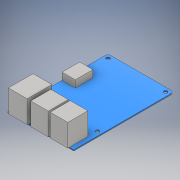
# Autodesk Inventor part: learnbotOdroid
Saved by Autodesk Inventor 2017 (Build 210142000, 142)
## iProperties
Part Number: learnbotOdroid
Material: Genérico
Document SubType Name: Modeling
Designer: rober
Density: 1 g/cm^3
Appearance: Valor por defecto
Author: rober
Autodesk Inventor part; units mm, degrees
ref_plane "YZ Plane" through (0, 0, 0) normal (1, 0, 0) x (0, 1, 0)
ref_plane "XZ Plane" through (0, 0, 0) normal (0, 1, 0) x (-1, 0, 0)
ref_plane "XY Plane" through (0, 0, 0) normal (0, 0, 1) x (1, 0, 0)
sketch "Boceto1" plane through (0, 0, 0) normal (0, 0, 1) x (1, 0, 0)
  line L0 (0.25, 8.5) -> (5.35, 8.5)
  line L1 (5.6, 8.25) -> (5.6, 0)
  line L2 (0, 0) -> (0, 8.25)
  line L3 (5.6, 0) -> (5.4774, 0)
  line L4 (0.18, -0.1368) -> (1.78, -0.1368)
  line L5 (2.09, -0.1465) -> (3.59, -0.1465)
  line L6 (3.74, -0.1465) -> (5.24, -0.1465)
  line L7 (0.18, 0) -> (0, 0)
  line L8 (2.09, 0) -> (1.78, 0)
  line L9 (3.59, 0) -> (3.74, 0)
  line L10 (5.24, 0) -> (5.6, 0)
  line L11 (1.1232, 4.6) -> (1.1232, 6.1)
  line L12 (1.1232, 6.1) -> (0, 6.1)
  line L13 (1.1232, 4.6) -> (0, 4.6)
  line L14 (0, 8.25) -> (0, 8.15)
  circle A0 centre (0.35, 8.15) radius 0.15
  circle A1 centre (5.25, 8.15) radius 0.15
  circle A2 centre (0.35, 2.35) radius 0.15
  circle A3 centre (5.25, 2.35) radius 0.15
  arc A4 (0.25, 8.5) -> (0, 8.25) centre (0.25, 8.25) ccw
  arc A5 (5.6, 8.25) -> (5.35, 8.5) centre (5.35, 8.25) ccw
  line L15 (0, 0) -> (5.6, 0)
  constraints: 32 end point, 6 centre point, 4 point on circle, 4 point on line, 1 horizontal
extrude "Extrusión1" add sketch "Boceto1" against normal blind 0.1
sketch "Boceto2" plane through (0, 0, 0) normal (0, 0, 1) x (1, 0, 0)
  line L0 (0.25, 8.5) -> (5.35, 8.5)
  line L1 (5.6, 8.25) -> (5.6, 0)
  line L2 (0, 0) -> (0, 8.25)
  line L3 (5.6, 0) -> (5.4774, 0)
  line L4 (0.18, -0.1368) -> (1.78, -0.1368)
  line L5 (1.78, -0.1368) -> (1.78, 1.9632)
  line L6 (1.78, 1.9632) -> (0.18, 1.9632)
  line L7 (0.18, 1.9632) -> (0.18, -0.1368)
  line L8 (2.09, -0.1465) -> (3.59, -0.1465)
  line L9 (3.59, -0.1465) -> (3.59, 1.5535)
  line L10 (3.59, 1.5535) -> (2.09, 1.5535)
  line L11 (2.09, 1.5535) -> (2.09, -0.1465)
  line L12 (3.74, -0.1465) -> (5.24, -0.1465)
  line L13 (5.24, -0.1465) -> (5.24, 1.5535)
  line L14 (5.24, 1.5535) -> (3.74, 1.5535)
  line L15 (3.74, 1.5535) -> (3.74, -0.1465)
  line L16 (0.18, 0) -> (0, 0)
  line L17 (2.09, 0) -> (1.78, 0)
  line L18 (3.59, 0) -> (3.74, 0)
  line L19 (5.24, 0) -> (5.6, 0)
  line L20 (1.1232, 4.6) -> (1.1232, 6.1)
  line L21 (1.1232, 6.1) -> (0, 6.1)
  line L22 (1.1232, 4.6) -> (0, 4.6)
  line L23 (0, 8.25) -> (0, 8.15)
  circle A0 centre (0.35, 8.15) radius 0.15
  circle A1 centre (5.25, 8.15) radius 0.15
  circle A2 centre (0.35, 2.35) radius 0.15
  circle A3 centre (5.25, 2.35) radius 0.15
  arc A4 (0.25, 8.5) -> (0, 8.25) centre (0.25, 8.25) ccw
  arc A5 (5.6, 8.25) -> (5.35, 8.5) centre (5.35, 8.25) ccw
  constraints: 48 end point, 10 point on line, 6 centre point, 4 point on circle
extrude "Extrusión2" add sketch "Boceto2" along normal blind 1.9 contours L13 L12 L15 L14 | L7 L6 L5 L4 | L9 L8 L11 L10
sketch "Boceto3" plane through (0, 0, 0) normal (0, 0, 1) x (1, 0, 0)
  line L0 (0.25, 8.5) -> (5.35, 8.5)
  line L1 (5.6, 8.25) -> (5.6, 0)
  line L2 (0, 0) -> (0, 8.25)
  line L3 (5.6, 0) -> (5.4774, 0)
  line L4 (0.18, -0.1368) -> (1.78, -0.1368)
  line L5 (1.78, -0.1368) -> (1.78, 1.9632)
  line L6 (1.78, 1.9632) -> (0.18, 1.9632)
  line L7 (0.18, 1.9632) -> (0.18, -0.1368)
  line L8 (2.09, -0.1465) -> (3.59, -0.1465)
  line L9 (3.59, -0.1465) -> (3.59, 1.5535)
  line L10 (3.59, 1.5535) -> (2.09, 1.5535)
  line L11 (2.09, 1.5535) -> (2.09, -0.1465)
  line L12 (3.74, -0.1465) -> (5.24, -0.1465)
  line L13 (5.24, -0.1465) -> (5.24, 1.5535)
  line L14 (5.24, 1.5535) -> (3.74, 1.5535)
  line L15 (3.74, 1.5535) -> (3.74, -0.1465)
  line L16 (0.18, 0) -> (0, 0)
  line L17 (2.09, 0) -> (1.78, 0)
  line L18 (3.59, 0) -> (3.74, 0)
  line L19 (5.24, 0) -> (5.6, 0)
  line L20 (1.1232, 4.6) -> (1.1232, 6.1)
  line L21 (1.1232, 6.1) -> (0, 6.1)
  line L22 (1.1232, 4.6) -> (0, 4.6)
  line L23 (0, 8.25) -> (0, 8.15)
  circle A0 centre (0.35, 8.15) radius 0.15
  circle A1 centre (5.25, 8.15) radius 0.15
  circle A2 centre (0.35, 2.35) radius 0.15
  circle A3 centre (5.25, 2.35) radius 0.15
  arc A4 (0.25, 8.5) -> (0, 8.25) centre (0.25, 8.25) ccw
  arc A5 (5.6, 8.25) -> (5.35, 8.5) centre (5.35, 8.25) ccw
  point P0 (0, 0)
  constraints: 48 end point, 10 point on line, 6 centre point, 4 point on circle
extrude "Extrusión3" add sketch "Boceto3" along normal blind 0.6 contours L21 L20 L22 L2
